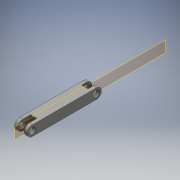
# Autodesk Inventor part: ArmSpan
Saved by Autodesk Inventor 2016 (Build 200138000, 138)
## iProperties
Created: 2016-11-02
Part Number: ArmSpan
Material: Generic
Document SubType Name: Modeling
Designer: mattc
Density: 1 g/cm^3
Appearance: Smooth - Medium Gray
Author: mattc
Autodesk Inventor part; units mm, degrees
ref_plane "YZ Plane" through (0, 0, 0) normal (1, 0, 0) x (0, 1, 0)
ref_plane "XZ Plane" through (0, 0, 0) normal (0, 1, 0) x (-1, 0, 0)
ref_plane "XY Plane" through (0, 0, 0) normal (0, 0, 1) x (1, 0, 0)
sketch "Sketch1" plane through (0, 0, 0) normal (1, 0, 0) x (0, 1, 0)
  circle A0 centre (0, 0) radius 2.5
  arc A1 (0, 4) -> (0, -4) centre (0, 0) ccw
  line L0 (0, 4) -> (50, 4)
  line L1 (50, -4) -> (0, -4)
  arc A2 (50, -4) -> (50, 4) centre (50, 0) ccw
  circle A3 centre (50, 0) radius 2.5
  dimension "d0" = 5
  dimension "d1" = 8
  dimension "d3" = 50
  dimension "d5" = 5
  dimension "d26" = 4
  constraints: 4 centre point, 4 end point, 4 point on circle, 3 coincident, 3 tangent, 1 horizontal, 1 parallel
  measures "d0" diameter of A0
  measures "d1" diameter of A1
  measures "d3" distance of L0.start L0.end
  measures "d5" diameter of A3
  measures "d26" radius of A2
extrude "Extrusion1" add sketch "Sketch1" along normal blind 10
ref_plane "Work Plane1" through (5, 0, 0) normal (1, 0, 0) x (0, 0, -1)
sketch "Sketch6" plane through (5, 0, 0) normal (1, 0, 0) x (0, 0, -1)
  line L0 (-4, 50) -> (-4, 0) projected
  line L1 (-4, 6) -> (4, 6)
  line L2 (4, 6) -> (4, -4)
  line L3 (4, -4) -> (-4, -4)
  line L4 (-4, -4) -> (-4, 6)
  line L5 (-4, 46) -> (4, 46)
  line L6 (4, 46) -> (4, 54)
  line L7 (4, 54) -> (-4, 54)
  line L8 (-4, 54) -> (-4, 46)
  circle A0 centre (0, 50) radius 2.5 projected
  point P0 (0, 0)
  dimension "d32" = 8
  dimension "d33" = 10
  dimension "d34" = 4
  dimension "d35" = 8
  dimension "d36" = 8
  dimension "d37" = 4
  dimension "d38" = 4
  constraints: 16 end point, 4 parallel, 2 horizontal, 2 perpendicular, 1 point on line
  measures "d32" distance of L2.end L3.end
  measures "d33" distance of L1.end L2.end
  measures "d34" distance from line of point (0, 0) L3
  measures "d35" distance of L7.end L6.end
  measures "d36" distance of L6.end L5.end
  measures "d37" distance from line of L5 A0.centre
  measures "d38" distance from line of L8 A0.centre
extrude "Extrusion5" cut sketch "Sketch6" along normal mid plane 5
equation "\"d5\" = d0"
equation "\"d26\" = 0.5 * d1"
equation "\"d34\" = 0.5 * d32"
equation "\"d35\" = d32"
equation "\"d36\" = d32"
equation "\"d37\" = 0.5 * d32"
equation "\"d38\" = 0.5 * d32"
body "Solid1"
